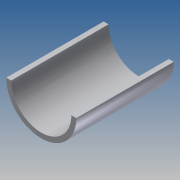
# Autodesk Inventor part: sparSplit2_5
Saved by Autodesk Inventor 2014 SP1 (Build 180222100, 222)
## iProperties
Created: 2014-09-04
Part Number: sparSplit2_5
Material: PVC-Piping
Document SubType Name: Modeling
Designer: Dave
Mass: 78.1883 g
Surface Area: 238.099 cm^2
Volume: 55.8488 cm^3
Density: 1.4 g/cm^3
Appearance: Smooth - White
Author: Dave
Autodesk Inventor part; units mm, degrees
ref_plane "YZ Plane" through (0, 0, 0) normal (1, 0, 0) x (0, 1, 0)
ref_plane "XZ Plane" through (0, 0, 0) normal (0, 1, 0) x (-1, 0, 0)
ref_plane "XY Plane" through (0, 0, 0) normal (0, 0, 1) x (1, 0, 0)
sketch "Sketch1" plane through (0, 0, 0) normal (0, 0, 1) x (1, 0, 0)
  arc A0 (-36.5125, 0) -> (36.5125, 0) centre (0, 0) ccw
  arc A1 (-31.3563, 0) -> (31.3563, 0) centre (0, 0) ccw
  line L0 (-36.5125, 0) -> (-31.3563, 0)
  line L1 (31.3563, 0) -> (36.5125, 0)
  dimension "d0" = 73.025
  dimension "d1" = 5.1562
  constraints: 4 end point, 4 point on circle, 2 centre point, 2 horizontal, 1 coincident
  measures "d0" diameter of A0
  measures "d1" radial gap between concentric circles of A1 A0
extrude "Extrusion1" add sketch "Sketch1" along normal blind 101.6
body "Solid1"
